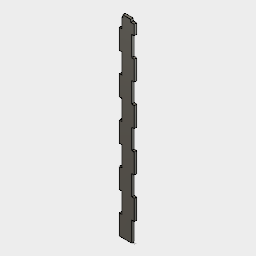
pillar v1 (Autodesk Fusion 360 design; units mm, degrees)
Autodesk Fusion 360 part; units mm, degrees
sketch "スケッチ1" plane through (0, 0, 0) normal (0, 0, 1) x (1, 0, 0)
  line L0 (20.0472, -16.9044) -> (20.0472, -26.9043)
  line L1 (20.0472, -26.9043) -> (17.5473, -26.9043)
  line L2 (17.5473, -26.9043) -> (17.5473, -46.9043)
  line L3 (17.5473, -46.9043) -> (20.0472, -46.9043)
  line L4 (20.0472, -46.9043) -> (20.0472, -66.9043)
  line L5 (20.0472, -66.9043) -> (17.5473, -66.9043)
  line L6 (17.5473, -66.9043) -> (17.5473, -86.9043)
  line L7 (17.5473, -86.9043) -> (20.0472, -86.9043)
  line L8 (20.0472, -86.9043) -> (20.0472, -106.9043)
  line L9 (20.0472, -106.9043) -> (17.5473, -106.9043)
  line L10 (17.5473, -106.9043) -> (17.5473, -126.9043)
  line L11 (17.5473, -126.9043) -> (20.0472, -126.9043)
  line L12 (20.0472, -126.9043) -> (20.0472, -146.9043)
  line L13 (20.0472, -146.9043) -> (17.5473, -146.9043)
  line L14 (17.5473, -146.9043) -> (17.5473, -166.9043)
  line L15 (17.5473, -166.9043) -> (20.0472, -166.9043)
  line L16 (20.0472, -166.9043) -> (20.0472, -186.9045)
  line L17 (20.0472, -186.9045) -> (17.5473, -186.9045)
  line L18 (17.5473, -186.9045) -> (17.5473, -206.9043)
  spline S0 degree 3 poles (17.5473, -206.9043) (17.5473, -206.9046) (30.0472, -206.9046) (30.0473, -206.9046) knots 19 19 19 19 20 20 20 20
  line L19 (30.0473, -206.9046) -> (30.0473, -186.9045)
  line L20 (30.0473, -186.9045) -> (32.5472, -186.9045)
  line L21 (32.5472, -186.9045) -> (32.5472, -166.9043)
  line L22 (32.5472, -166.9043) -> (30.0473, -166.9043)
  line L23 (30.0473, -166.9043) -> (30.0473, -146.9043)
  line L24 (30.0473, -146.9043) -> (32.5472, -146.9043)
  line L25 (32.5472, -146.9043) -> (32.5472, -126.9043)
  line L26 (32.5472, -126.9043) -> (30.0473, -126.9043)
  line L27 (30.0473, -126.9043) -> (30.0473, -106.9043)
  line L28 (30.0473, -106.9043) -> (32.5472, -106.9043)
  line L29 (32.5472, -106.9043) -> (32.5472, -86.9043)
  line L30 (32.5472, -86.9043) -> (30.0473, -86.9043)
  line L31 (30.0473, -86.9043) -> (30.0473, -66.9043)
  line L32 (30.0473, -66.9043) -> (32.5472, -66.9043)
  line L33 (32.5472, -66.9043) -> (32.5472, -46.9043)
  line L34 (32.5472, -46.9043) -> (30.0473, -46.9043)
  line L35 (30.0473, -46.9043) -> (30.0473, -26.9043)
  line L36 (30.0473, -26.9043) -> (32.5472, -26.9043)
  line L37 (32.5472, -26.9043) -> (32.5472, -16.9044)
  line L38 (32.5472, -16.9044) -> (29.0473, -16.9044)
  line L39 (29.0473, -16.9044) -> (29.0473, -14.4045)
  line L40 (29.0473, -14.4045) -> (21.0473, -14.4045)
  line L41 (21.0473, -14.4045) -> (21.0473, -16.9044)
  line L42 (21.0473, -16.9044) -> (20.0472, -16.9044)
extrude "押し出し1" add sketch "スケッチ1" along normal blind 2.5
